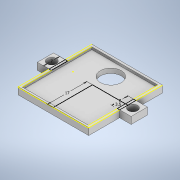
# Autodesk Inventor part: sheel
Saved by Autodesk Inventor 2020.2 (Build 242310000, 310)
## iProperties
Created: 2020-02-10
Part Number: sheel
Material: Generic
Document SubType Name: Modeling
Designer: ColinP
Density: 1 g/cm^3
Appearance: Default
Author: ColinP
Autodesk Inventor part; units mm, degrees
ref_plane "YZ Plane" through (0, 0, 0) normal (1, 0, 0) x (0, 1, 0)
ref_plane "XZ Plane" through (0, 0, 0) normal (0, 1, 0) x (-1, 0, 0)
ref_plane "XY Plane" through (0, 0, 0) normal (0, 0, 1) x (1, 0, 0)
sketch "Sketch1" plane through (0, 0, 0) normal (0, 1, 0) x (-1, 0, 0)
  line L0 (6.29, 17.6429) -> (-24.19, 17.6429)
  line L1 (-24.19, 17.6429) -> (-24.19, -14.3571)
  line L2 (-24.19, -14.3571) -> (6.29, -14.3571)
  line L3 (6.29, -14.3571) -> (6.29, 17.6429)
  point P0 (0, 0)
  dimension "d0" = 30.48
  dimension "d1" = 32
  constraints: 8 end point, 3 perpendicular, 1 horizontal
  measures "d0" distance of L0.start L0.end
  measures "d1" distance of L0.end L1.end
extrude "Extrusion1" add sketch "Sketch1" along normal blind 2
sketch "Sketch3" plane through (0, 2, 0) normal (0, 1, 0) x (1, 0, 0)
  line L0 (-6.29, -17.6429) -> (24.19, -17.6429) projected
  line L1 (-6.29, -17.6429) -> (-6.29, -16.6429)
  line L2 (-6.29, 14.3571) -> (-6.29, -17.6429) projected
  line L3 (-6.29, -16.6429) -> (-5.29, -16.6429)
  line L4 (-5.29, -16.6429) -> (-5.29, 13.3571)
  line L5 (24.19, 14.3571) -> (-6.29, 14.3571) projected
  line L6 (24.19, -17.6429) -> (24.19, 14.3571) projected
  line L7 (24.19, -17.6429) -> (23.19, -17.6429)
  line L8 (23.19, -17.6429) -> (23.19, -16.6429)
  line L9 (23.19, -16.6429) -> (23.19, 3.3571)
  line L10 (23.19, -16.6429) -> (-5.29, -16.6429)
  line L11 (-5.29, -16.6429) -> (-5.29, 13.3571)
  line L12 (-5.29, 13.3571) -> (23.19, 13.3571)
  line L13 (23.19, 13.3571) -> (23.19, -16.6429)
  point P0 (0, 0)
  dimension "d4" = 1
  dimension "d5" = 1
  dimension "d6" = 30
  dimension "d7" = 1
  constraints: 20 end point, 4 perpendicular, 3 point on line, 2 parallel, 1 horizontal
  measures "d4" distance of L0.start L1.end
  measures "d5" distance of L1.end L3.end
  measures "d6" distance of L3.end L4.end
  measures "d7" distance of L0.end L7.end
extrude "Extrusion3" add sketch "Sketch3" along normal blind 1 contours L1 L3 L10 L8 L0 | L8 L9 L13 L12 L4 L3 L2 L5 L6 L0
sketch "Sketch4" plane through (0, 0, 0) normal (0, -1, 0) x (1, 0, 0)
  line L0 (24.19, -14.3571) -> (-6.29, -14.3571) projected
  line L1 (8.95, -14.3571) -> (8.95, -7.3571)
  point P0 (0, 0)
  dimension "d12" = 7
  constraints: 2 end point, 1 midpoint, 1 vertical
  measures "d12" distance of L1.start L1.end
hole "Hole1" at (8.95, 0, -7.3571) direction (0, 1, 0) diameter 9 end through all
sketch "Sketch5" plane through (0, 3, 0) normal (0, 1, 0) x (1, 0, 0)
  line L0 (-6.29, -17.6429) -> (24.19, -17.6429) projected
  line L1 (8.95, -17.6429) -> (8.95, -0.6429)
  line L2 (8.95, -0.6429) -> (24.19, -0.6429)
  line L3 (24.19, -17.6429) -> (24.19, 14.3571) projected
  line L4 (24.19, -0.6429) -> (24.19, -4.1429)
  line L5 (24.19, -4.1429) -> (23.19, -4.1429)
  line L6 (23.19, -16.6429) -> (23.19, 13.3571) projected
  line L7 (23.19, -4.1429) -> (23.19, 2.8571)
  line L8 (23.19, 2.8571) -> (24.19, 2.8571)
  line L9 (24.19, 2.8571) -> (24.19, -4.1429)
  line L10 (-5.29, -16.6429) -> (-5.29, 13.3571) projected
  line L11 (-5.29, -0.6429) -> (-5.29, -4.1429)
  line L12 (-5.29, -4.1429) -> (-6.29, -4.1429)
  line L13 (-6.29, 14.3571) -> (-6.29, -17.6429) projected
  line L14 (-6.29, -4.1429) -> (-6.29, 2.8571)
  line L15 (-6.29, 2.8571) -> (-5.29, 2.8571)
  line L16 (-5.29, -0.6429) -> (-5.29, 2.8571)
  point P0 (0, 0)
  dimension "d20" = 17
  dimension "d21" = 3.5
  dimension "d22" = 7
  dimension "d23" = 7
  constraints: 24 end point, 13 point on line, 4 perpendicular, 2 vertical, 1 collinear, 1 midpoint
  measures "d20" distance of L1.start L1.end
  measures "d21" distance of L2.end L4.end
  measures "d22" distance of L5.end L7.end
  measures "d23" distance of L12.end L14.end
sketch "Sketch6" plane through (0, 0, 0) normal (0, -1, 0) x (1, 0, 0)
  line L0 (-5.29, 4.1429) -> (-6.29, 4.1429) projected
  line L1 (-6.29, -2.8571) -> (-5.29, -2.8571) projected
  line L2 (23.19, -2.8571) -> (24.19, -2.8571) projected
  line L3 (24.19, 4.1429) -> (23.19, 4.1429) projected
  line L4 (-5.29, -13.3571) -> (-5.29, 16.6429) projected
  line L5 (-6.29, -14.3571) -> (-6.29, 17.6429) projected
  line L6 (23.19, 16.6429) -> (23.19, -13.3571) projected
  line L7 (24.19, 17.6429) -> (24.19, -14.3571) projected
  line L8 (24.19, 4.1429) -> (29.19, 4.1429)
  line L9 (29.19, 4.1429) -> (29.19, -2.8571)
  line L10 (29.19, -2.8571) -> (24.19, -2.8571)
  line L11 (-6.29, -2.8571) -> (-11.29, -2.8571)
  line L12 (-11.29, -2.8571) -> (-11.29, 4.1429)
  line L13 (-11.29, 4.1429) -> (-6.29, 4.1429)
  point P0 (0, 0)
  dimension "d26" = 5
  dimension "d27" = 5
  constraints: 12 end point, 4 perpendicular, 2 point on line, 1 horizontal
  measures "d26" distance of L3.start L8.end
  measures "d27" distance of L1.start L11.end
extrude "Extrusion5" add sketch "Sketch6" against normal blind 3 contours L5 L11 L12 L13 | L7 L8 L9 L10
sketch "Sketch7" plane through (0, 0, 0) normal (0, -1, 0) x (1, 0, 0)
  line L0 (-6.29, 17.6429) -> (24.19, 17.6429) projected
  line L1 (8.95, 17.6429) -> (8.95, 0.6429)
  line L2 (8.95, 0.6429) -> (26.45, 0.6429)
  line L3 (26.45, 0.6429) -> (-8.55, 0.6429)
  point P0 (0, 0)
  dimension "d30" = 17
  dimension "d31" = 17.5
  dimension "d32" = 35
  constraints: 6 end point, 1 midpoint, 1 perpendicular, 1 point on line, 1 vertical
  measures "d30" distance of L1.start L1.end
  measures "d31" distance of L1.end L2.end
  measures "d32" distance of L2.end L3.end
hole "Hole2" at (-8.55, 0, 0.6429) at (26.45, 0, 0.6429) direction (0, 1, 0) diameter 4 end through all
sketch "Sketch8" plane through (-6.29, 0, 17.6429) normal (0, 0, 1) x (1, 0, 0)
  line L0 (0, 0) -> (0, 3) projected
  line L1 (1, 3) -> (0, 3) projected
  line L2 (1, 3) -> (1, 3.5) projected
  line L3 (0, 3.5) -> (1, 3.5) projected
  line L4 (-5, 0) -> (-5, 3.25) projected
  line L5 (0, 0) -> (-5, 0) projected
  line L6 (0, 3) -> (0, 0) projected
  line L7 (0, 0) -> (30.48, 0) projected
  line L8 (30.48, 0) -> (30.48, 3) projected
  line L9 (0, 3) -> (30.48, 3) projected
  line L10 (0, 0) -> (0, 3) projected
  line L11 (0, 3.25) -> (0, 3.5) projected
  line L12 (-5, 3.25) -> (0, 3.25) projected
  point P0 (6.29, 0)
extrude "Extrusion6" cut sketch "Sketch8" against normal blind 0.2 contours L0 L1 L9 L8 L7
body "Solid1"
